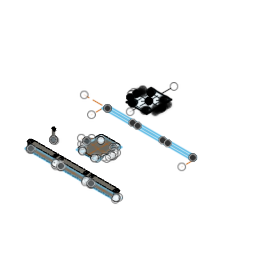
Multi FS40 Bracket v35 (Autodesk Fusion 360 design; units mm, degrees)
Autodesk Fusion 360 part; units mm, degrees
note: some values were not read from the file. Chosen so that the rebuilt part matches the saved one: which face or edge a step refers to. Set by a fixed rule: which sketch regions a step uses.
sketch "Schizzo1" plane through (0, 0, 0) normal (0, 0, 1) x (1, 0, 0)
  line L0 (32, -39) -> (-32, -39)
  line L1 (-32, -39) -> (-32, 39)
  line L2 (-32, 39) -> (32, 39)
  line L3 (32, 39) -> (32, -39)
  line L4 (32, -39) -> (-32, 39) construction
  line L5 (-32, -39) -> (32, 39) construction
  line L6 (-19.25, 24.7) -> (19.25, 24.7) construction
  line L7 (19.25, 24.7) -> (19.25, -33.8) construction
  line L8 (19.25, -33.8) -> (-19.25, -33.8) construction
  line L9 (-19.25, -33.8) -> (-19.25, 24.7) construction
  circle A0 centre (-19.25, 24.7) radius 1.7
  line L10 (0, 0) -> (0, 80) construction
  line L11 (0, 0) -> (0, -60) construction
  line L12 (-32, 0) -> (32, 0) construction
  circle A1 centre (-19.25, -33.8) radius 1.7
  circle A2 centre (19.25, -33.8) radius 1.7
  circle A3 centre (19.25, 24.7) radius 1.7
  line L13 (-32, 0) -> (-48, 0) construction
  line L14 (-40, 20.7498) -> (-40, -19.8726) construction
  circle A4 centre (-40, 0) radius 8
  line L15 (-40, -8) -> (-46, -8) construction
  line L16 (-46, -11.1) -> (-32, -11.1) construction
  arc A5 (-32, -11.1) -> (-40, -8) centre (-40, -19.8726) ccw
  arc A6 (-40, 8) -> (-32, 11.1) centre (-40, 19.8726) ccw
  circle A7 centre (40, 0) radius 8
  arc A8 (32, 11.1) -> (40, 8) centre (40, 19.8726) ccw
  arc A9 (40, -8) -> (32, -11.1) centre (40, -19.8726) ccw
  line L17 (-53.5, -78.6928) -> (226.9, -78.6928)
  line L18 (226.9, -78.6928) -> (226.9, -94.6928)
  line L19 (226.9, -94.6928) -> (-53.5, -94.6928)
  line L20 (-53.5, -94.6928) -> (-53.5, -78.6928)
  circle A10 centre (-45.5, -86.6928) radius 8
  line L21 (-45.5, -78.6928) -> (-45.5, -94.6928) construction
  circle A11 centre (-45.5, -86.6928) radius 2.9
  line L22 (34.5, -78.6928) -> (34.5, -94.6928) construction
  line L23 (226.9, -86.6928) -> (-120, -86.6928) construction
  circle A12 centre (34.5, -86.6928) radius 2.9
  line L24 (50.7, -78.6928) -> (50.7, -94.6928) construction
  circle A13 centre (50.7, -86.6928) radius 2.9
  line L25 (130.7, -78.6928) -> (130.7, -94.6928) construction
  circle A14 centre (130.7, -86.6928) radius 2.9
  line L26 (146.9, -78.6928) -> (146.9, -94.6928) construction
  line L27 (226.9, -78.6928) -> (226.9, -94.6928) construction
  circle A15 centre (146.9, -86.6928) radius 2.9
  circle A16 centre (226.9, -86.6928) radius 2.9
  circle A17 centre (226.9, -86.6928) radius 8
  line L28 (-53.5, -86.6928) -> (234.9, -86.6928)
  line L29 (234.9, -86.6928) -> (-53.5, -86.6928)
  line L30 (-53.5, -86.6928) -> (-53.5, -130) construction
  line L31 (234.9, -86.6928) -> (234.9, -130) construction
  circle A18 centre (-40, 0) radius 3.1
  circle A19 centre (40, 0) radius 3.1
  circle A20 centre (-22, -29) radius 10
  circle A21 centre (22, -29) radius 10
  circle A22 centre (-22, 29) radius 10
  circle A23 centre (22, 29) radius 10
  line L32 (20, -171.9) -> (84, -171.9)
  line L33 (84, -171.9) -> (84, -249.9)
  line L34 (84, -249.9) -> (20, -249.9)
  line L35 (20, -249.9) -> (20, -171.9)
  line L36 (20, -210.9) -> (84, -210.9) construction
  circle A24 centre (12, -210.9) radius 3.2
  line L37 (12, -210.9) -> (12, -202.9) construction
  circle A25 centre (12, -207.7) radius 3.2
  line L38 (8.8, -207.7) -> (8.8, -210.9)
  line L39 (15.2, -210.9) -> (15.2, -207.7)
  line L40 (15.2, -210.9) -> (8.8, -210.9) construction
  circle A26 centre (12, -210.9) radius 8
  line L41 (12, -202.9) -> (20, -202.9) construction
  line L42 (20, -202.9) -> (20, -194.9)
  line L43 (20, -194.9) -> (12, -194.9) construction
  line L44 (12, -194.9) -> (12, -202.9) construction
  arc A27 (12, -202.9) -> (20, -194.9) centre (12, -194.9) ccw
  arc A28 (20, -226.9) -> (12, -218.9) centre (12, -226.9) ccw
  line L45 (52, -171.9) -> (52, -249.9) construction
  circle A29 centre (92, -210.9) radius 8
  circle A30 centre (92, -210.9) radius 3.2
  circle A31 centre (92, -207.7) radius 3.2
  line L46 (95.2, -207.7) -> (95.2, -210.9)
  line L47 (88.8, -210.9) -> (88.8, -207.7)
  arc A32 (92, -218.9) -> (84, -226.9) centre (92, -226.9) ccw
  arc A33 (84, -194.9) -> (92, -202.9) centre (92, -194.9) ccw
  circle A34 centre (28, -241.9) radius 8
  circle A35 centre (76, -241.9) radius 8
  circle A36 centre (76, -179.9) radius 8
  circle A37 centre (28, -179.9) radius 8
  line L48 (71.25, -186.2) -> (32.75, -186.2) construction
  line L49 (32.75, -186.2) -> (32.75, -244.7) construction
  line L50 (32.75, -244.7) -> (71.25, -244.7) construction
  line L51 (71.25, -244.7) -> (71.25, -186.2) construction
  line L52 (52, -186.2) -> (52, -244.7) construction
  line L53 (71.25, -215.45) -> (32.75, -215.45) construction
  circle A38 centre (71.25, -186.2) radius 1.7
  circle A39 centre (32.75, -186.2) radius 1.7
  circle A40 centre (71.25, -244.7) radius 1.7
  circle A41 centre (32.75, -244.7) radius 1.7
  circle A42 centre (39.4992, -320.5305) radius 3.1
  line L54 (42.5992, -317.4305) -> (39.4992, -317.4305)
  line L55 (39.4992, -320.5305) -> (39.4992, -317.4305) construction
  line L56 (39.4992, -320.5305) -> (36.3992, -320.5305) construction
  line L57 (42.5992, -323.6305) -> (39.4992, -323.6305)
  line L58 (39.4992, -317.4305) -> (43.2, -317.4305) construction
  line L59 (43.2, -323.6305) -> (39.4992, -323.6305) construction
  line L60 (39.4992, -323.6305) -> (39.4992, -317.4305) construction
  circle A43 centre (42.5992, -320.5305) radius 3.1
  line L61 (127.4992, -312.5305) -> (31.4992, -312.5305)
  line L62 (31.4992, -312.5305) -> (31.4992, -328.5305)
  line L63 (31.4992, -328.5305) -> (127.4992, -328.5305)
  line L64 (127.4992, -328.5305) -> (127.4992, -312.5305)
  line L65 (127.4992, -320.5305) -> (31.4992, -320.5305) construction
  circle A44 centre (119.4992, -320.5305) radius 8
  circle A45 centre (39.4992, -320.5305) radius 8
  line L66 (43.7053, -313.7254) -> (43.7053, -327.3356) construction
  line L67 (12, -207.7) -> (8.8, -207.7) construction
  line L68 (12, -207.7) -> (15.2, -207.7) construction
  line L69 (20, -210.9) -> (-5, -210.9) construction
  circle A46 centre (39.4992, -320.5305) radius 6.2
  circle A47 centre (39.4992, -320.5305) radius 4.1
  circle A48 centre (12, -210.9) radius 4.1
  circle A49 centre (92, -210.9) radius 4.1
  line L70 (36.4992, -312.5305) -> (36.4992, -328.5305) construction
  line L71 (36.4992, -315.1046) -> (36.4992, -325.9564)
  line L72 (79.4992, -312.5305) -> (79.4992, -328.5305) construction
  circle A50 centre (119.4992, -320.5305) radius 6.2
  circle A51 centre (116.3992, -320.5305) radius 3.1
  circle A52 centre (119.4992, -320.5305) radius 4.1
  circle A53 centre (119.4992, -320.5305) radius 3.1
  line L73 (122.4992, -315.1046) -> (122.4992, -325.9564)
  line L74 (138.7992, -317.4305) -> (135.6992, -317.4305)
  line L75 (175.6992, -312.5305) -> (175.6992, -328.5305) construction
  circle A54 centre (135.6992, -320.5305) radius 4.1
  line L76 (138.7992, -323.6305) -> (135.6992, -323.6305)
  line L77 (223.6992, -320.5305) -> (127.6992, -320.5305) construction
  circle A55 centre (135.6992, -320.5305) radius 8
  circle A56 centre (215.6992, -320.5305) radius 4.1
  line L78 (223.6992, -328.5305) -> (223.6992, -312.5305)
  line L79 (223.6992, -312.5305) -> (127.6992, -312.5305)
  circle A57 centre (212.5992, -320.5305) radius 3.1
  line L80 (135.6992, -323.6305) -> (135.6992, -317.4305) construction
  circle A58 centre (135.6992, -320.5305) radius 3.1
  line L81 (135.6992, -320.5305) -> (135.6992, -317.4305) construction
  line L82 (132.6992, -315.1046) -> (132.6992, -325.9564)
  line L83 (135.6992, -317.4305) -> (139.4, -317.4305) construction
  line L84 (139.9053, -313.7254) -> (139.9053, -327.3356) construction
  line L85 (127.6992, -328.5305) -> (223.6992, -328.5305)
  circle A59 centre (138.7992, -320.5305) radius 3.1
  line L86 (218.6992, -315.1046) -> (218.6992, -325.9564)
  line L87 (132.6992, -312.5305) -> (132.6992, -328.5305) construction
  line L88 (139.4, -323.6305) -> (135.6992, -323.6305) construction
  circle A60 centre (215.6992, -320.5305) radius 8
  circle A61 centre (215.6992, -320.5305) radius 6.2
  line L89 (135.6992, -320.5305) -> (132.5992, -320.5305) construction
  circle A62 centre (135.6992, -320.5305) radius 6.2
  circle A63 centre (215.6992, -320.5305) radius 3.1
  line L90 (127.6992, -312.5305) -> (127.6992, -328.5305)
  line L91 (-52.4947, -313.7254) -> (-52.4947, -327.3356) construction
  circle A64 centre (-56.7008, -320.5305) radius 4.1
  line L92 (-53.6008, -317.4305) -> (-56.7008, -317.4305)
  line L93 (-53.6008, -323.6305) -> (-56.7008, -323.6305)
  line L94 (31.2992, -312.5305) -> (-64.7008, -312.5305)
  circle A65 centre (-53.6008, -320.5305) radius 3.1
  circle A66 centre (23.2992, -320.5305) radius 3.1
  line L95 (-56.7008, -317.4305) -> (-53, -317.4305) construction
  line L96 (-59.7008, -312.5305) -> (-59.7008, -328.5305) construction
  line L97 (-64.7008, -328.5305) -> (31.2992, -328.5305)
  line L98 (-53, -323.6305) -> (-56.7008, -323.6305) construction
  line L99 (26.2992, -315.1046) -> (26.2992, -325.9564)
  line L100 (-56.7008, -320.5305) -> (-59.8008, -320.5305) construction
  line L101 (-64.7008, -312.5305) -> (-64.7008, -328.5305)
  line L102 (31.2992, -320.5305) -> (-64.7008, -320.5305) construction
  line L103 (-56.7008, -320.5305) -> (-56.7008, -317.4305) construction
  circle A67 centre (20.1992, -320.5305) radius 3.1
  circle A68 centre (23.2992, -320.5305) radius 4.1
  line L104 (-16.7008, -312.5305) -> (-16.7008, -328.5305) construction
  circle A69 centre (23.2992, -320.5305) radius 6.2
  line L105 (-59.7008, -315.1046) -> (-59.7008, -325.9564)
  circle A70 centre (23.2992, -320.5305) radius 8
  line L106 (31.2992, -328.5305) -> (31.2992, -312.5305)
  line L107 (-56.7008, -323.6305) -> (-56.7008, -317.4305) construction
  line L108 (31.4992, -312.5305) -> (31.4992, -328.5305)
  circle A71 centre (-56.7008, -320.5305) radius 6.2
  circle A72 centre (-56.7008, -320.5305) radius 3.1
  circle A73 centre (-56.7008, -320.5305) radius 8
  line L109 (-64.7008, -312.5305) -> (223.6992, -312.5305)
  line L110 (223.6992, -312.5305) -> (223.6992, -328.5305)
  line L111 (223.6992, -328.5305) -> (-64.7008, -328.5305)
  line L112 (-64.7008, -328.5305) -> (-64.7008, -312.5305)
  circle A74 centre (71.25, -186.2) radius 3
  circle A75 centre (32.75, -186.2) radius 3
  circle A76 centre (71.25, -244.7) radius 3
  circle A77 centre (32.75, -244.7) radius 3
  line L113 (-41, -260.6) -> (-49, -260.6)
  line L114 (-49, -260.6) -> (-49, -259.4)
  line L115 (-49, -259.4) -> (-41, -259.4)
  line L116 (-49, -260.6) -> (-41, -259.4) construction
  circle A78 centre (-45, -260) radius 4
  line L117 (-41, -260.6) -> (-49, -259.4) construction
  line L118 (-43, -260.6) -> (-43, -261.5)
  line L119 (-40.4019, -260) -> (-43, -261.5)
  line L120 (-43, -259.4) -> (-43, -258.5)
  line L121 (-51, -260) -> (-39, -260) construction
  line L122 (-41, -259.4) -> (-41, -260.6)
  line L123 (-43, -256.5359) -> (-43, -263.4641) construction
  line L124 (-40.4019, -260) -> (-43, -258.5)
  circle A79 centre (-45, -260) radius 6
  point P0 (32.75, -186.2)
  point P1 (-45, -260)
  dimension "d1" = 64
  dimension "d2" = 78
  dimension "d3" = 33.8
  dimension "d5" = 58.5
  dimension "d6" = 19.25
  dimension "d7" = 38.5
  dimension "d8" = 3.4
  dimension "d9" = 3.4
  dimension "d17" = 8
  dimension "d18" = 16
  dimension "d19" = 3.1
  dimension "d20" = 80
  dimension "d21" = 16
  dimension "d22" = 8
  dimension "d23" = 5.8
  dimension "d24" = 80
  dimension "d25" = 5.8
  dimension "d28" = 96.2
  dimension "d29" = 5.8
  dimension "d30" = 80
  dimension "d32" = 5.8
  dimension "d33" = 96.2
  dimension "d34" = 80
  dimension "d35" = 5.8
  dimension "d36" = 5.8
  dimension "d39" = 6.2
  dimension "d87" = 10
  dimension "d88" = 288.4
  dimension "d106" = 64
  dimension "d107" = 78
  dimension "d108" = 6.4
  dimension "d112" = 16
  dimension "d113" = 8
  dimension "d114" = 8
  dimension "d115" = 8
  dimension "d116" = 38.5
  dimension "d117" = 58.5
  dimension "d118" = 3.4
  dimension "d119" = 33.8
  dimension "d122" = 6.2
  dimension "d124" = 96
  dimension "d125" = 16
  dimension "d134" = 12.4
  dimension "d139" = 8.2
  dimension "d142" = 8.2
  dimension "d143" = 3
  dimension "d144" = 80
  dimension "d165" = 6.2
  dimension "d166" = 96
  dimension "d167" = 16
  dimension "d168" = 12.4
  dimension "d169" = 8.2
  dimension "d170" = 3
  dimension "d171" = 80
  dimension "d172" = 6.2
  dimension "d173" = 96
  dimension "d174" = 16
  dimension "d175" = 12.4
  dimension "d176" = 8.2
  dimension "d177" = 3
  dimension "d178" = 80
  dimension "d186" = 6
  dimension "d190" = 12
  dimension "d191" = 8
  dimension "d192" = 8
  dimension "d193" = 1.2
  dimension "d194" = 2
  dimension "d195" = 30
  constraint horizontal L0
  constraint perpendicular L0 L1
  constraint parallel L0 L2
  constraint parallel L1 L3
  constraint coincident L4 L10.start
  constraint coincident L5 L10.start
  constraint coincident L10.start L11.start
  constraint horizontal L6
  constraint vertical L7
  constraint horizontal L8
  constraint vertical L9
  constraint coincident L6.start L9.end
  constraint perpendicular L2 L10
  constraint perpendicular L0 L11
  constraint midpoint L1 L12.start
  constraint midpoint L3 L12.end
  constraint coincident L8.end L9.start
  constraint symmetric A0 L11 A3
  constraint symmetric L11 A1 A2
  constraint perpendicular L1 L13
  constraint vertical L14
  constraint coincident A4 L15.start
  constraint coincident L14 L15.start
  constraint tangent A4 L15
  constraint horizontal L16
  constraint coincident L1 L16.end
  constraint coincident L14 A5.centre
  constraint symmetric L13 L15.start A6.start
  constraint symmetric L13 L16.end A6.end
  constraint symmetric L13 A5 A6
  constraint symmetric L10 A4 A7
  constraint symmetric L10 L15.start A9.start
  constraint symmetric L10 L16.end A9.end
  constraint symmetric L10 A5 A9
  constraint symmetric L10 A6.end A8.start
  constraint symmetric L10 A6.start A8.end
  constraint symmetric L10 A6 A8
  constraint horizontal L17
  constraint vertical L18
  constraint horizontal L19
  constraint vertical L20
  constraint tangent L20 A10
  constraint tangent L19 A10
  constraint perpendicular L17 L21
  constraint coincident A10.centre L21
  constraint concentric A10 A11
  constraint perpendicular L19 L22
  constraint midpoint L18 L23.start
  constraint perpendicular L21 L23
  constraint coincident L22 A12.centre
  constraint coincident L23 A12.centre
  constraint perpendicular L19 L24
  constraint coincident L24 A13.centre
  constraint coincident L23 A13.centre
  constraint perpendicular L19 L25
  constraint coincident L25 A14.centre
  constraint coincident L23 A14.centre
  constraint perpendicular L19 L26
  constraint perpendicular L19 L27
  constraint coincident L26 A15.centre
  constraint coincident L23 A15.centre
  constraint coincident L27 L23.start
  constraint coincident L23 A16.centre
  constraint concentric A16 A17
  constraint tangent L17 A17
  constraint midpoint L20 L28.start
  constraint coincident A17 L28.end
  constraint coincident L23 L28.end
  constraint tangent A10 L30
  constraint perpendicular L28 L30
  constraint tangent A17 L31
  constraint coincident L14.end A5.centre
  constraint coincident L13 A4.centre
  constraint concentric A4 A18
  constraint symmetric L10 A18 A19
  constraint tangent L1 A20
  constraint tangent L0 A20
  constraint symmetric L11 A20 A21
  constraint symmetric L12 A20 A22
  constraint symmetric L12 A21 A23
  constraint horizontal L32
  constraint vertical L33
  constraint horizontal L34
  constraint vertical L35
  constraint midpoint L35 L36.start
  constraint midpoint L33 L36.end
  constraint coincident A24.centre L37.start
  constraint perpendicular L32 L37
  constraint coincident L37 A25.centre
  constraint vertical L38
  constraint vertical L39
  constraint tangent A24 L39
  constraint coincident A24 L39.start
  constraint coincident A24 L38.end
  constraint horizontal L40
  constraint coincident L39.start L40.start
  constraint collinear L36 L40
  constraint coincident L36 A24.centre
  constraint tangent L35 A26
  constraint coincident L37.end A26
  constraint horizontal L41
  constraint vertical L42
  constraint horizontal L43
  constraint vertical L44
  constraint tangent L35 A27
  constraint symmetric L36 L37.end A28.end
  constraint symmetric L36 L42.end A28.start
  constraint symmetric L36 A27 A28
  constraint midpoint L32 L45.start
  constraint midpoint L34 L45.end
  constraint symmetric A24 L45 A30
  constraint symmetric L37.end L45 A33.end
  constraint symmetric A25 L45 A31
  constraint symmetric L39.end L45 L47.end
  constraint symmetric L38.start L45 L46.start
  constraint symmetric L38.end L45 L46.end
  constraint symmetric L39.start L45 L47.start
  constraint symmetric A26 L45 A29
  constraint symmetric L42.end L45 A33.start
  constraint symmetric A27 L45 A33
  constraint symmetric A28.end L45 A32.start
  constraint symmetric A28.start L45 A32.end
  constraint symmetric A28 L45 A32
  constraint tangent L34 A34
  constraint tangent L35 A34
  constraint symmetric L45 A34 A35
  constraint symmetric L36 A34 A37
  constraint symmetric L36 A35 A36
  constraint horizontal L48
  constraint vertical L49
  constraint horizontal L50
  constraint vertical L51
  constraint midpoint L48 L52.start
  constraint midpoint L50 L52.end
  constraint midpoint L51 L53.start
  constraint midpoint L49 L53.end
  constraint coincident L48.start L51.end
  constraint symmetric L48.start L52 P0
  constraint symmetric L52 A38 A39
  constraint symmetric L53 A38 A40
  constraint symmetric L53 A39 A41
  constraint collinear L45 L52
  constraint horizontal L54
  constraint tangent A42 L54
  constraint coincident A42.centre L55.start
  constraint coincident A42 L54.end
  constraint vertical L55
  constraint coincident A42 L56.end
  constraint perpendicular L55 L56
  constraint coincident L54.end L55.end
  constraint symmetric L54.start L56 L57.start
  constraint symmetric L54.end L56 L57.end
  constraint horizontal L58
  constraint horizontal L59
  constraint vertical L60
  constraint coincident L57 L59.start
  constraint tangent L54 A43
  constraint tangent L57 A43
  constraint coincident L54.start A43
  constraint horizontal L61
  constraint vertical L62
  constraint horizontal L63
  constraint vertical L64
  constraint midpoint L64 L65.start
  constraint midpoint L62 L65.end
  constraint collinear L56 L65
  constraint tangent L61 A44
  constraint tangent L64 A44
  constraint tangent L63 A44
  constraint tangent L63 A45
  constraint tangent L62 A45
  constraint tangent L61 A45
  constraint coincident A45 L66.start
  constraint coincident A45 L66.end
  constraint perpendicular L63 L66
  constraint tangent L60 A43
  constraint coincident L38 L40.end
  constraint coincident A24.centre A25
  constraint tangent A25 L38
  constraint coincident A25.centre L67.start
  constraint coincident A25 L38.start
  constraint tangent A24 L67
  constraint perpendicular L37 L67
  constraint coincident A25 L39.end
  constraint tangent A24 L68
  constraint parallel L67 L68
  constraint coincident L38.start L67.end
  constraint coincident L38.end L40.end
  constraint coincident L39.end L68.end
  constraint perpendicular L35 L69
  constraint concentric A42 A47
  constraint concentric A24 A48
  constraint symmetric L45 A48 A49
  constraint coincident L61 L70.start
  constraint coincident L63 L70.end
  constraint perpendicular L63 L70
  constraint coincident A46 L71.start
  constraint coincident L70 L71.start
  constraint coincident A46 L71.end
  constraint coincident L70 L71.end
  constraint midpoint L61 L72.start
  constraint midpoint L63 L72.end
  constraint symmetric A42 L72 A53
  constraint symmetric A43 L72 A51
  constraint symmetric A46 L72 A50
  constraint symmetric A47 L72 A52
  constraint symmetric L71.start L72 L73.start
  constraint symmetric L71.end L72 L73.end
  constraint horizontal L74
  constraint tangent L74 A58
  constraint coincident A54.centre A55.centre
  constraint coincident L74.end A58
  constraint vertical L81
  constraint coincident L89.end A58
  constraint perpendicular L81 L89
  constraint coincident L74.end L80.end
  constraint symmetric L76.start L74.start L89
  constraint symmetric L76.end L74.end L89
  constraint horizontal L83
  constraint horizontal L88
  constraint vertical L80
  constraint coincident L88.start L76
  constraint tangent L74 A59
  constraint tangent L76 A59
  constraint coincident L74.start A59
  constraint horizontal L79
  constraint vertical L90
  constraint horizontal L85
  constraint vertical L78
  constraint midpoint L77.start L78
  constraint midpoint L77.end L90
  constraint collinear L77 L89
  constraint tangent L79 A60
  constraint tangent L78 A60
  constraint tangent L85 A60
  constraint tangent A55 L85
  constraint tangent A55 L90
  constraint tangent A55 L79
  constraint coincident L84.start A55
  constraint coincident L84.end A55
  constraint perpendicular L84 L85
  constraint tangent L80 A59
  constraint concentric A54 A58
  constraint coincident L87.start L79
  constraint coincident L87.end L85
  constraint perpendicular L85 L87
  constraint coincident L82.start A62
  constraint coincident L82.start L87
  constraint coincident L82.end A62
  constraint coincident L82.end L87
  constraint midpoint L75.start L79
  constraint midpoint L75.end L85
  constraint symmetric L75 A58 A63
  constraint symmetric L75 A57 A59
  constraint symmetric L75 A61 A62
  constraint symmetric L75 A54 A56
  constraint symmetric L86.start L82.start L75
  constraint symmetric L86.end L82.end L75
  constraint horizontal L92
  constraint tangent L92 A72
  constraint coincident A64.centre L100.start
  constraint coincident L92.end A72
  constraint vertical L103
  constraint coincident L100.end A72
  constraint perpendicular L100 L103
  constraint coincident L92.end L95.start
  constraint symmetric L93.start L92.start L100
  constraint symmetric L93.end L92.end L100
  constraint horizontal L95
  constraint horizontal L98
  constraint vertical L107
  constraint coincident L98.start L93
  constraint tangent L92 A65
  constraint tangent L93 A65
  constraint coincident L92.start A65
  constraint horizontal L94
  constraint vertical L101
  constraint horizontal L97
  constraint vertical L106
  constraint midpoint L102.start L106
  constraint midpoint L102.end L101
  constraint collinear L100 L102
  constraint tangent L94 A70
  constraint tangent A70 L106
  constraint tangent L97 A70
  constraint tangent L97 A73
  constraint tangent L101 A73
  constraint tangent L94 A73
  constraint coincident L91.start A73
  constraint coincident L91.end A73
  constraint perpendicular L91 L97
  constraint tangent A65 L107
  constraint concentric A64 A72
  constraint coincident L96.start L94
  constraint coincident L96.end L97
  constraint perpendicular L96 L97
  constraint coincident L105.start A71
  constraint coincident L105.start L96
  constraint coincident L105.end A71
  constraint coincident L105.end L96
  constraint midpoint L104.start L94
  constraint midpoint L104.end L97
  constraint symmetric A66 L104 A72
  constraint symmetric A65 A67 L104
  constraint symmetric L104 A69 A71
  constraint symmetric A64 A68 L104
  constraint symmetric L99.start L105.start L104
  constraint symmetric L99.end L105.end L104
  constraint vertical L108
  constraint horizontal L109
  constraint vertical L110
  constraint horizontal L111
  constraint vertical L112
  constraint concentric A38 A74
  constraint symmetric L45 A74 A75
  constraint symmetric L53 A74 A76
  constraint symmetric L53 A75 A77
  constraint concentric A78 A79
  constraint horizontal L113
  constraint perpendicular L113 L114
  constraint parallel L113 L115
  constraint parallel L114 L122
  constraint coincident P1 L117
  constraint coincident P1 L116
  constraint coincident P1 A78.centre
  constraint coincident L123.start A78
  constraint coincident L123.end A78
  constraint vertical L123
  constraint coincident L121.start A79
  constraint coincident L121.end A79
  constraint parallel L115 L121
  constraint coincident L119.start L121
  constraint coincident L120.end L123
  constraint coincident L120.start L115
  constraint coincident L120.start L123
  constraint perpendicular L115 L120
  constraint symmetric L119.start L124.start L121
  constraint symmetric L120.end L118.end L121
  constraint symmetric L120.start L118.start L121
  constraint coincident L17 L21.start
  constraint coincident L17 L22.start
  constraint coincident L17 L24.start
  constraint coincident L17 L25.start
  constraint coincident L17 L26.start
  constraint coincident L17.end A17
  constraint coincident L19 L24.end
  constraint coincident L19 L25.end
  constraint coincident L19 L22.end
  constraint coincident L19 L21.end
  constraint coincident L19 L26.end
  measures "d1" distance of L1.end L2.end
  measures "d2" distance of L0.end L1.end
  measures "d3" distance of L10.start L8
  measures "d5" distance of L6 L8
  measures "d6" distance of L10.start L9
  measures "d7" distance of L7 L9
  measures "d8" diameter of A0
  measures "d9" diameter of A1
  measures "d17" distance of L1 L14.start
  measures "d18" diameter of A4
  measures "d19" distance of L15 L16
  measures "d20" distance of L14 A7.centre
  measures "d21" distance of L17.start L19.end
  measures "d22" radius of A10
  measures "d23" diameter of A11
  measures "d24" distance of L21 L22
  measures "d25" diameter of A12
  measures "d28" distance of A10.centre L24
  measures "d29" diameter of A13
  measures "d30" distance of L24 L25
  measures "d32" diameter of A14
  measures "d33" distance of L24 L26.end
  measures "d34" distance of L26 L27
  measures "d35" diameter of A15
  measures "d36" diameter of A16
  measures "d39" diameter of A18
  measures "d87" radius of A20
  measures "d88" distance of L30 L31
  measures "d106" distance of L33.end L34.end
  measures "d107" distance of L32 L34
  measures "d108" diameter of A24
  measures "d112" diameter of A26
  measures "d113" distance of L37.end L41.end
  measures "d114" distance of L37.end L43.end
  measures "d115" radius of A34
  measures "d116" distance of L48.start P0
  measures "d117" distance of L48.start L50.end
  measures "d118" diameter of A38
  measures "d119" distance of L36 L50
  measures "d122" diameter of A42
  measures "d124" distance of L61.start L61.end
  measures "d125" distance of L61.start L63.end
  measures "d134" diameter of A46
  measures "d139" diameter of A47
  measures "d142" diameter of A48
  measures "d143" distance of L60 L70
  measures "d144" distance of A42.centre A44.centre
  measures "d165" diameter of A58
  measures "d166" distance of L78.end L79.end
  measures "d167" distance of L78.start L78.end
  measures "d168" diameter of A62
  measures "d169" diameter of A54
  measures "d170" distance of L80 L87
  measures "d171" distance of A56.centre A54.centre
  measures "d172" diameter of A72
  measures "d173" distance of L94.start L94.end
  measures "d174" distance of L97.end L94.start
  measures "d175" diameter of A71
  measures "d176" diameter of A64
  measures "d177" distance of L96 L107
  measures "d178" distance of A66.centre A64.centre
  measures "d186" diameter of A74
  measures "d190" diameter of A79
  measures "d191" diameter of A78
  measures "d192" distance of L114.end L115.end
  measures "d193" distance of L114.end L113.end
  measures "d194" distance of L122 L123
  measures "d195" angle of L121 L124
extrude "Estrusione1" add sketch "Schizzo1" along normal blind 4 contours L0 L1 L2 L3 A20 A21 A22 A23 | A21 | A20 | L3 A7 A9 | L3 A7 A8 | A7 | L1 A4 A5 | L1 A4 A6 | A4 | A23 | A22 makes body 1
pattern_linear "Serie R1" count 1 spacing 0 along (0, 1, 0) count 3 spacing 96.2 along (1, 0, 0) of bodies 1 makes body 2 at (102.3333, 0.3426, 0) makes body 3 at (198.5333, 0.3426, 0)
extrude "Estrusione2" add sketch "Schizzo1" along normal blind 20 separate body contours L17 A10 A12 A13 A14 A15 A17 L28 L29 | A10 A11 L28 L29 | A10 A11 L28 L29 | L18 A16 A17 L28 L29 | L18 A16 A17 L28 L29 | L19 A10 A12 A13 A14 A15 A17 L28 L29 | L18 A16 A17 L28 L29 | L18 A16 A17 L28 L29 makes body 4
extrude "Estrusione16" add sketch "Schizzo1" along normal blind 5 separate body contours L32 L33 L34 L35 L42 A34 A35 A36 A37 A74 A75 A76 A77 | A37 A75 | A36 A74 | L35 A26 L42 A27 | A37 A39 A75 | A37 A39 A75 | A36 A38 A74 | A36 A38 A74 | A26 | L33 A29 A33 | L35 A26 A28 | L33 A29 A32 | A29 | A34 A77 | A35 A76 | A35 A76 | A35 A76 | A34 A77 | A34 A77 makes body 5
extrude "Estrusione26" cut sketch "Schizzo1" along normal blind 3.2 from surface at 1.8 contours A37 A39 A75 | A37 A39 A75 | A36 A38 A74 | A36 A38 A74 | A35 A76 | A35 A76 | A34 A77 | A34 A77 picked at (68.8429, -244.5366) picked at (68.7431, -245.6171) picked at (34.7512, -246.4676) picked at (35.1571, -244.5366) bodies 5
extrude "Estrusione17" add sketch "Schizzo1" along normal blind 20 separate body contours A42 A43 | A42 A43 A47 | A42 A43 L71 | A42 L54 A43 A47 | A42 L57 A43 A47 | A42 L54 A47 L71 | L54 A43 A47 | A43 A47 | A42 L57 A47 L71 | L57 A43 A47 | A42 L71 | A42 A47 L71 | L54 A43 A46 A47 L71 | L57 A43 A46 A47 L71 | A46 A47 L71 | L61 L63 A44 A45 L109 L111 | A44 | A45 | A50 A52 L73 | A50 A51 A52 L73 | A50 A51 A52 L73 | A51 A52 | A51 A52 A53 L73 | A52 A53 L73 | A51 A52 A53 L73 | A51 A52 A53 | A51 A53 L73 | A53 L73 | A51 A53 makes body 6
extrude "Estrusione18" cut sketch "Schizzo1" along normal blind 20 contours A42 A43 | A42 A43 A47 | A42 A43 L71 | A42 L54 A43 A47 | A42 L57 A43 A47 | A42 L54 A47 L71 | L54 A43 A47 | A43 A47 | A42 L57 A47 L71 | L57 A43 A47 | A42 L71 | A42 A47 L71 | A51 A52 | A51 A52 A53 L73 | A52 A53 L73 | A51 A52 A53 L73 | A51 A52 A53 | A51 A53 L73 | A53 L73 | A51 A53 bodies 6
extrude "Estrusione19" cut sketch "Schizzo1" along normal blind 4 from surface at 16 contours A42 A43 A47 | A42 L54 A43 A47 | A42 L57 A43 A47 | A42 L54 A47 L71 | L54 A43 A47 | A43 A47 | A42 L57 A47 L71 | L57 A43 A47 | A42 A47 L71 | L54 A43 A46 A47 L71 | L57 A43 A46 A47 L71 | A50 A51 A52 L73 | A50 A51 A52 L73 | A52 A53 L73 bodies 6
pattern_linear "Serie R3" count 3 spacing 96.2 along (1, 0, 0) both ways of "Estrusione17", "Estrusione18", "Estrusione19" makes body 7 at (-3.3675, -312.5305, 6.6667) makes body 8 at (189.0325, -312.5305, 6.6667)
extrude "Estrusione25" add sketch "Schizzo1" along normal blind 20 contours L61 L64 A44 L109 | L64 L90 L109 L111 | L63 L64 A44 L111 | A55 L79 L90 L109 | L61 L62 A45 L108 L109 | A55 L85 L90 L111 | L62 L106 L108 L109 L111 | L62 L63 A45 L108 L111 | L94 A70 L106 L109 | L97 A70 L106 L111 bodies 6 7 8
extrude "Estrusione27" add sketch "Schizzo1" along normal blind 7 separate body contours L113 A78 L119 L122 | L113 A78 L118 L119 | L113 A78 L119 | L119 L122 L124 | A78 L119 L122 | L113 L118 L119 | L113 L115 A78 L119 L124 | L113 L114 A78 | A78 L122 L124 | L114 L115 A78 | L115 A78 L122 L124 | L115 A78 L124 | L115 A78 L120 L124 | L115 L120 L124 | A79 makes body 9
extrude "Estrusione28" cut sketch "Schizzo1" along normal blind 2 contours L119 L122 L124 | L113 L118 L119 | L113 L115 A78 L119 L124 | L115 L120 L124 bodies 9
extrude "Estrusione29" add sketch "Schizzo1" along normal blind 21 from surface at 7 contours L113 A78 L118 L119 | L113 A78 L119 | L113 L118 L119 | L113 L115 A78 L119 L124 | L115 A78 L124 | L115 A78 L120 L124 | L115 L120 L124 bodies 9
sketch "Schizzo10" plane through (0, 0, 28) normal (0, 0, 1) x (-1, 0, 0)
  circle A0 centre (45, 260) radius 4
  line L0 (45, 257) -> (45, 263) construction
  line L1 (39, 263) -> (48, 263) construction
  line L2 (42, 257) -> (42, 263) construction
  line L3 (45, 263) -> (42, 263)
  line L4 (45, 257) -> (42, 257) construction
  line L5 (39, 257) -> (39, 263) construction
  arc A1 (42, 263) -> (42, 257) centre (42, 260) ccw
  line L6 (48, 257) -> (39, 257) construction
  line L7 (45, 257) -> (42, 257)
  line L8 (48, 257) -> (45, 257) construction
  arc A2 (45, 257) -> (45, 263) centre (45, 260) ccw
  line L9 (48, 263) -> (48, 257) construction
  line L10 (42, 257) -> (39, 257) construction
  circle A3 centre (45, 260) radius 4
  line L11 (48, 260) -> (39, 260) construction
  line L12 (41, 260.6) -> (49, 260.6) construction
  line L13 (49, 260.6) -> (49, 259.4) construction
  line L14 (49, 259.4) -> (41, 259.4) construction
  line L15 (41, 259.4) -> (41, 260.6) construction
  line L16 (41, 260.6) -> (49, 259.4) construction
  line L17 (49, 260.6) -> (41, 259.4) construction
  line L18 (43, 256.5359) -> (43, 263.4641) construction
  line L19 (43, 258.55) -> (40.4885, 260)
  line L20 (43, 258.55) -> (40.1, 258.55) construction
  line L21 (48, 260) -> (48, 259.4)
  line L22 (48, 259.4) -> (43, 259.4)
  line L23 (43, 259.4) -> (43, 258.55)
  line L24 (48, 260) -> (48, 260.6)
  line L25 (43, 260.6) -> (43, 261.45)
  line L26 (43, 261.45) -> (40.4885, 260)
  line L27 (48, 260.6) -> (43, 260.6)
  point P0 (45, 260)
  point P1 (45, 260)
  point P2 (45, 260)
  dimension "d209" = 9
  dimension "d210" = 6
  dimension "d211" = 8
  dimension "d212" = 1.2
  dimension "d214" = 2
  dimension "d215" = 30
  constraint horizontal L6
  constraint vertical L5
  constraint horizontal L1
  constraint vertical L9
  constraint midpoint L11.start L9
  constraint midpoint L11.end L5
  constraint coincident L0.start L6
  constraint coincident L0.end L1
  constraint perpendicular L0 L1
  constraint coincident L2.start L6
  constraint coincident L2.end L1
  constraint perpendicular L1 L2
  constraint equal L8 L10
  constraint equal L4 L8
  constraint midpoint P2 L0
  constraint midpoint A1.centre L2
  constraint coincident P2 P1
  constraint horizontal L12
  constraint perpendicular L12 L13
  constraint parallel L12 L14
  constraint parallel L13 L15
  constraint coincident L16 P2
  constraint coincident L17 P2
  constraint coincident A3 L18.start
  constraint coincident A3 L18.end
  constraint perpendicular L1 L18
  constraint horizontal L20
  constraint coincident L18 L19.start
  constraint coincident L11 L19.end
  constraint coincident L9 L21.end
  constraint coincident L14 L21.end
  constraint coincident L18 L22.end
  constraint coincident L14 L22.end
  constraint symmetric L21.start L11 L24.start
  constraint symmetric L11 L19.start L25.end
  constraint symmetric L11 L19.end L26.end
  constraint symmetric L11 L21.end L24.end
  constraint symmetric L11 L22.end L25.start
  measures "d209" distance of L6.start L5.start
  measures "d210" distance of L6.start L1.end
  measures "d211" distance of L13.end L14.end
  measures "d212" distance of L12.end L13.end
  measures "d214" distance of L15 L18
  measures "d215" angle of L19 L20
extrude "Estrusione30" add sketch "Schizzo10" along normal blind 4 bodies 9
extrude "Estrusione31" cut sketch "Schizzo10" along normal blind 2 from surface at 2 contours A0 A2 A3 L19 L22 L23 L25 L26 L27 | A0 A3 L19 L26 bodies 9
hidden bodies 1 2 3 4
equation "d6 = 38.50 mm / 2"
named bodies: "Basetta 1", "Basetta 2", "Basetta 3", "Trave", "BasettaQDS-1", "TraveQDS", "TraveQDS (1)", "TraveQDS (2)", "Mounting Screw V3"
